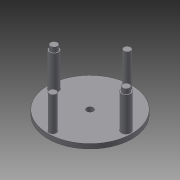
# Autodesk Inventor part: 1005
Saved by Autodesk Inventor 2015 (Build 190159000, 159)
## iProperties
Created: 2015-10-05
Part Number: 1005
Material: 一般
Document SubType Name: シート メタル
Designer: kenta
Density: 1 g/cm^3
Sheet Metal Rule: Default_mm
Appearance: 既定
Author: kenta
Autodesk Inventor part; units mm, degrees
ref_plane "YZ Plane" through (0, 0, 0) normal (1, 0, 0) x (0, 1, 0)
ref_plane "XZ Plane" through (0, 0, 0) normal (0, 1, 0) x (-1, 0, 0)
ref_plane "XY Plane" through (0, 0, 0) normal (0, 0, 1) x (1, 0, 0)
sketch "スケッチ1" plane through (0, 0, 0) normal (0, 0, 1) x (1, 0, 0)
  circle A0 centre (0, 0) radius 18
  dimension "d0" = 36
  constraints: 1 centre point, 1 coincident
  measures "d0" diameter of A0
extrude "押し出し1" add sketch "スケッチ1" along normal blind 2
sketch "スケッチ2" plane through (0, 0, 2) normal (0, 0, 1) x (1, 0, 0)
  circle A0 centre (-15.5, 0) radius 2
  circle A1 centre (15.5, 0) radius 2
  point P0 (0, 0)
  dimension "d3" = 4
  dimension "d4" = 4
  dimension "d5" = 0
  dimension "d6" = 0
  dimension "d8" = 15.5
  dimension "d9" = 31
  constraints: 2 centre point
  measures "d3" diameter of A1
  measures "d4" diameter of A0
  measures "d5" vertical distance of A0.centre A1.centre
  measures "d6" vertical distance of point (0, 0) A1.centre
  measures "d8" distance of point (0, 0) A1.centre
  measures "d9" distance of A1.centre A0.centre
extrude "押し出し2" add sketch "スケッチ2" along normal blind 14.5
sketch "スケッチ3" plane through (-15.5, 0, 16.5) normal (0, 0, 1) x (1, 0, 0)
  circle A0 centre (0, 0) radius 1.5
  circle A1 centre (31, 0) radius 1.5
  circle A2 centre (0, 0) radius 2 projected
  point P0 (15.5, 0)
  dimension "d12" = 3
  dimension "d13" = 3
  dimension "d14" = 31
  dimension "d15" = 0
  constraints: 2 centre point
  measures "d12" diameter of A1
  measures "d13" diameter of A0
  measures "d14" distance of A1.centre A0.centre
  measures "d15" distance of A2.centre A0.centre
extrude "押し出し3" add sketch "スケッチ3" along normal blind 2 contours A0 | A1
sketch "スケッチ4" plane through (0, 0, 2) normal (0, 0, 1) x (1, 0, 0)
  circle A0 centre (0, 16) radius 1.5
  circle A1 centre (0, -16) radius 1.5
  point P0 (0, 0)
  dimension "d18" = 3
  dimension "d19" = 3
  dimension "d20" = 32
  dimension "d21" = 16
  constraints: 2 centre point
  measures "d18" diameter of A1
  measures "d19" diameter of A0
  measures "d20" distance of A0.centre A1.centre
  measures "d21" distance of point (0, 0) A1.centre
extrude "押し出し4" add sketch "スケッチ4" along normal blind 14.5
sketch "スケッチ5" plane through (0, 0, 2) normal (0, 0, 1) x (1, 0, 0)
  circle A0 centre (0, 0) radius 1.4
  dimension "d24" = 2.8
  constraints: 1 centre point, 1 coincident
  measures "d24" diameter of A0
extrude "押し出し5" cut sketch "スケッチ5" against normal blind 3
equation "\"BendRadius\" = Thickness"
equation "\"BendReliefWidth\" = Thickness"
equation "\"BendReliefDepth\" = 0.5 * Thickness"
equation "\"CornerReliefSize\" = 4 * Thickness"
equation "\"MinimumRemnant\" = 2 * Thickness"
equation "\"TransitionRadius\" = BendRadius"
equation "\"JacobiRadiusSize\" = BendRadius"
equation "\"GapSize\" = Thickness"
equation "\"Thickness\" = 0.5"
